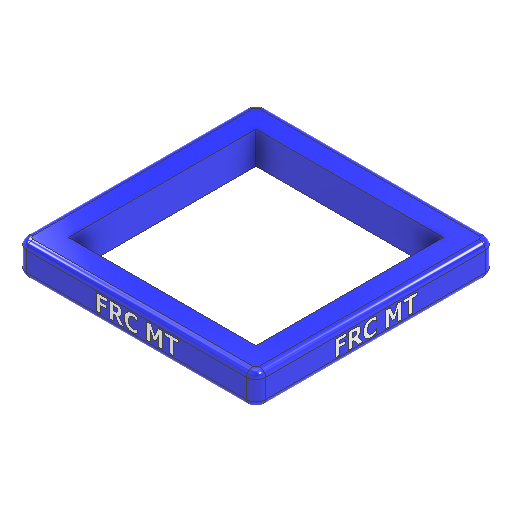
# Autodesk Inventor part: Bumper
Saved by Autodesk Inventor 2025.3 (Build 293356000, 356)
## iProperties
Created: 2026-05-15
Part Number: Bumper
Material: Genérico
Document SubType Name: Modeling
Designer: djair.oliveira
Density: 1 g/cm^3
Appearance: Padrão
Author: djair.oliveira
Autodesk Inventor part; units mm, degrees
ref_plane "YZ Plane" through (0, 0, 0) normal (1, 0, 0) x (0, 1, 0)
ref_plane "XZ Plane" through (0, 0, 0) normal (0, 1, 0) x (-1, 0, 0)
ref_plane "XY Plane" through (0, 0, 0) normal (0, 0, 1) x (1, 0, 0)
sketch "Esboço1" plane through (0, 0, 0) normal (0, 1, 0) x (-1, 0, 0)
  line L0 (-292.1, 292.1) -> (292.1, 292.1)
  line L1 (292.1, 292.1) -> (292.1, -292.1)
  line L2 (292.1, -292.1) -> (-292.1, -292.1)
  line L3 (-292.1, -292.1) -> (-292.1, 292.1)
  line L4 (-292.1, 292.1) -> (292.1, -292.1) construction
  line L5 (292.1, 292.1) -> (-292.1, -292.1) construction
  line L6 (-342.1, 372.1) -> (342.1, 372.1)
  line L7 (372.1, 342.1) -> (372.1, -342.1)
  line L8 (342.1, -372.1) -> (-342.1, -372.1)
  line L9 (-372.1, -342.1) -> (-372.1, 342.1)
  line L10 (-372.1, 372.1) -> (372.1, -372.1) construction
  line L11 (372.1, 372.1) -> (-372.1, -372.1) construction
  arc A0 (-372.1, -342.1) -> (-342.1, -372.1) centre (-342.1, -342.1) ccw
  arc A1 (-342.1, 372.1) -> (-372.1, 342.1) centre (-342.1, 342.1) ccw
  arc A2 (372.1, 342.1) -> (342.1, 372.1) centre (342.1, 342.1) ccw
  arc A3 (342.1, -372.1) -> (372.1, -342.1) centre (342.1, -342.1) ccw
  point P0 (0, 0)
  dimension "d0" = 584.2
  dimension "d1" = 584.2
  dimension "d2" = 80
  dimension "d3" = 30
  constraints: 24 end point, 9 point on line, 8 point on circle, 8 tangent, 4 centre point, 4 midpoint, 4 parallel, 3 equal radius, 2 horizontal, 2 perpendicular
  measures "d0" distance of L0.end L1.end
  measures "d1" distance of L1.end L2.end
  measures "d2" distance between parallel lines of L9 L3
  measures "d3" radius of A0
extrude "Extrusão1" add sketch "Esboço1" along normal blind 100
fillet "Arredondamento1" radius 20 16 edges at (363.3132, 100, -363.3132) (0, 100, -372.1) (-363.3132, 100, -363.3132) (-372.1, 100, 0) (-363.3132, 100, 363.3132) (0, 100, 372.1) (363.3132, 100, 363.3132) (372.1, 100, 0) (363.3132, 0, -363.3132) (0, 0, -372.1) (-363.3132, 0, -363.3132) (-372.1, 0, 0) (-363.3132, 0, 363.3132) (0, 0, 372.1) (363.3132, 0, 363.3132) (372.1, 0, 0)
sketch "Esboço2" plane through (372.1, 20, -342.1) normal (1, 0, 0) x (0, 0, -1)
  line L0 (-513.8978, 55) -> (-170.3022, 55) construction
  line L1 (-170.3022, 55) -> (-170.3022, 5) construction
  line L2 (-170.3022, 5) -> (-513.8978, 5) construction
  line L3 (-513.8978, 5) -> (-513.8978, 55) construction
  line L4 (30, 0) -> (30, 60) projected
  line L5 (-433.1859, 44.5057) -> (-454.1746, 44.5057)
  line L6 (-454.1746, 44.5057) -> (-454.1746, 35.0648)
  line L7 (-454.1746, 35.0648) -> (-434.8472, 35.0648)
  line L8 (-434.8472, 35.0648) -> (-434.8472, 25.5429)
  line L9 (-434.8472, 25.5429) -> (-454.1746, 25.5429)
  line L10 (-454.1746, 25.5429) -> (-454.1746, 4.0276)
  line L11 (-454.1746, 4.0276) -> (-466.6543, 4.0276)
  line L12 (-466.6543, 4.0276) -> (-466.6543, 54.0276)
  line L13 (-466.6543, 54.0276) -> (-433.1859, 54.0276)
  line L14 (-433.1859, 54.0276) -> (-433.1859, 44.5057)
  line L15 (-380.5117, 4.0276) -> (-395.7872, 4.0276)
  line L16 (-395.7872, 4.0276) -> (-409.6851, 22.3825)
  line L17 (-409.6851, 22.3825) -> (-414.2232, 22.3825)
  line L18 (-414.2232, 22.3825) -> (-414.2232, 4.0276)
  line L19 (-414.2232, 4.0276) -> (-426.7029, 4.0276)
  line L20 (-426.7029, 4.0276) -> (-426.7029, 54.0276)
  line L21 (-426.7029, 54.0276) -> (-406.6057, 54.0276)
  spline S0 degree 2 poles (-406.6057, 54.0276) (-402.4322, 54.0276) (-396.2734, 52.9741) (-393.6397, 51.3533) knots 0 0 0 1 2 2 2
  spline S1 degree 2 poles (-393.6397, 51.3533) (-390.9655, 49.6515) (-387.805, 44.3436) (-387.805, 40.2917) knots 0 0 0 1 2 2 2
  spline S2 degree 2 poles (-387.805, 40.2917) (-387.805, 34.5786) (-392.9914, 27.4068) (-397.3269, 25.2998) knots 0 0 0 1 2 2 2
  line L22 (-397.3269, 25.2998) -> (-380.5117, 4.0276)
  spline S3 degree 2 poles (-400.6899, 38.7115) (-400.6899, 40.6159) (-402.1486, 43.3306) (-403.8099, 44.06) knots 0 0 0 1 2 2 2
  spline S4 degree 2 poles (-403.8099, 44.06) (-404.9849, 44.5462) (-407.8617, 44.8298) (-410.0092, 44.8298) knots 0 0 0 1 2 2 2
  line L23 (-410.0092, 44.8298) -> (-414.2232, 44.8298)
  line L24 (-414.2232, 44.8298) -> (-414.2232, 31.3776)
  line L25 (-414.2232, 31.3776) -> (-410.617, 31.3776)
  spline S5 degree 2 poles (-410.617, 31.3776) (-408.0238, 31.3776) (-404.3366, 32.0259) (-403.0805, 33.0389) knots 0 0 0 1 2 2 2
  spline S6 degree 2 poles (-403.0805, 33.0389) (-401.865, 34.0113) (-400.6899, 36.6045) (-400.6899, 38.7115) knots 0 0 0 1 2 2 2
  spline S7 degree 2 poles (-355.228, 3.0551) (-366.4922, 3.0551) (-379.7013, 16.6694) (-379.7013, 28.987) knots 0 0 0 1 2 2 2
  spline S8 degree 2 poles (-379.7013, 28.987) (-379.7013, 40.859) (-366.4517, 55) (-355.1875, 55) knots 0 0 0 1 2 2 2
  spline S9 degree 2 poles (-355.1875, 55) (-352.2297, 55) (-347.4485, 54.3112) (-345.2604, 53.7439) knots 0 0 0 1 2 2 2
  spline S10 degree 2 poles (-345.2604, 53.7439) (-343.5587, 53.2172) (-339.5473, 51.4749) (-338.2912, 50.8266) knots 0 0 0 1 2 2 2
  line L26 (-338.2912, 50.8266) -> (-338.2912, 38.9141)
  line L27 (-338.2912, 38.9141) -> (-339.5473, 38.9141)
  spline S11 degree 2 poles (-339.5473, 38.9141) (-340.4793, 39.7245) (-343.2345, 41.9935) (-344.9768, 43.047) knots 0 0 0 1 2 2 2
  spline S12 degree 2 poles (-344.9768, 43.047) (-346.7191, 44.141) (-350.8925, 45.6402) (-353.2021, 45.6402) knots 0 0 0 1 2 2 2
  spline S13 degree 2 poles (-353.2021, 45.6402) (-355.9169, 45.6402) (-360.4144, 43.9384) (-362.4809, 41.7909) knots 0 0 0 1 2 2 2
  spline S14 degree 2 poles (-362.4809, 41.7909) (-364.3447, 39.8865) (-366.7353, 33.363) (-366.7353, 28.9465) knots 0 0 0 1 2 2 2
  spline S15 degree 2 poles (-366.7353, 28.9465) (-366.7353, 24.2869) (-364.2637, 17.9254) (-362.2378, 15.9806) knots 0 0 0 1 2 2 2
  spline S16 degree 2 poles (-362.2378, 15.9806) (-360.2929, 14.0762) (-355.5117, 12.4149) (-353.1211, 12.4149) knots 0 0 0 1 2 2 2
  spline S17 degree 2 poles (-353.1211, 12.4149) (-350.6494, 12.4149) (-346.1519, 14.0762) (-344.6122, 15.0891) knots 0 0 0 1 2 2 2
  spline S18 degree 2 poles (-344.6122, 15.0891) (-342.9104, 16.1021) (-340.3577, 18.2496) (-339.4258, 19.1005) knots 0 0 0 1 2 2 2
  line L28 (-339.4258, 19.1005) -> (-338.2912, 19.1005)
  line L29 (-338.2912, 19.1005) -> (-338.2912, 7.3501)
  spline S19 degree 2 poles (-338.2912, 7.3501) (-339.6689, 6.7018) (-343.275, 5.081) (-345.2199, 4.5138) knots 0 0 0 1 2 2 2
  spline S20 degree 2 poles (-345.2199, 4.5138) (-347.57, 3.7844) (-351.6624, 3.0551) (-355.228, 3.0551) knots 0 0 0 1 2 2 2
  line L30 (-259.6851, 4.0276) -> (-272.1648, 4.0276)
  line L31 (-272.1648, 4.0276) -> (-272.1648, 37.1718)
  line L32 (-272.1648, 37.1718) -> (-281.241, 15.778)
  line L33 (-281.241, 15.778) -> (-289.831, 15.778)
  line L34 (-289.831, 15.778) -> (-298.9071, 37.1718)
  line L35 (-298.9071, 37.1718) -> (-298.9071, 4.0276)
  line L36 (-298.9071, 4.0276) -> (-310.7386, 4.0276)
  line L37 (-310.7386, 4.0276) -> (-310.7386, 54.0276)
  line L38 (-310.7386, 54.0276) -> (-296.2734, 54.0276)
  line L39 (-296.2734, 54.0276) -> (-285.1713, 29.3517)
  line L40 (-285.1713, 29.3517) -> (-274.1502, 54.0276)
  line L41 (-274.1502, 54.0276) -> (-259.6851, 54.0276)
  line L42 (-259.6851, 54.0276) -> (-259.6851, 4.0276)
  line L43 (-239.7094, 4.0276) -> (-239.7094, 44.5057)
  line L44 (-239.7094, 44.5057) -> (-254.4987, 44.5057)
  line L45 (-254.4987, 44.5057) -> (-254.4987, 54.0276)
  line L46 (-254.4987, 54.0276) -> (-212.3593, 54.0276)
  line L47 (-212.3593, 54.0276) -> (-212.3593, 44.5057)
  line L48 (-212.3593, 44.5057) -> (-227.1486, 44.5057)
  line L49 (-227.1486, 44.5057) -> (-227.1486, 4.0276)
  line L50 (-227.1486, 4.0276) -> (-239.7094, 4.0276)
  point P0 (-342.1, -20)
  point P1 (-342.1, 55)
  point P2 (-170.3022, 30)
  point P3 (30, 30)
  dimension "d12" = 50
  constraints: 3 midpoint, 1 horizontal, 1 horizontal alignment, 1 vertical alignment, 2 other
  measures "d12" distance of L0.end L1.end
extrude "Extrusão2" cut sketch "Esboço2" against normal blind 0.1
sketch "Esboço3" plane through (342.1, 20, -372.1) normal (0, 0, -1) x (-1, 0, 0)
  line L0 (136.9103, 55) -> (547.2897, 55) construction
  line L1 (547.2897, 55) -> (547.2897, 5) construction
  line L2 (547.2897, 5) -> (136.9103, 5) construction
  line L3 (136.9103, 5) -> (136.9103, 55) construction
  line L4 (714.2, 0) -> (714.2, 60) projected
  line L5 (251.0141, 44.5057) -> (230.0254, 44.5057)
  line L6 (230.0254, 44.5057) -> (230.0254, 35.0648)
  line L7 (230.0254, 35.0648) -> (249.3528, 35.0648)
  line L8 (249.3528, 35.0648) -> (249.3528, 25.5429)
  line L9 (249.3528, 25.5429) -> (230.0254, 25.5429)
  line L10 (230.0254, 25.5429) -> (230.0254, 4.0276)
  line L11 (230.0254, 4.0276) -> (217.5457, 4.0276)
  line L12 (217.5457, 4.0276) -> (217.5457, 54.0276)
  line L13 (217.5457, 54.0276) -> (251.0141, 54.0276)
  line L14 (251.0141, 54.0276) -> (251.0141, 44.5057)
  line L15 (303.6883, 4.0276) -> (288.4128, 4.0276)
  line L16 (288.4128, 4.0276) -> (274.5149, 22.3825)
  line L17 (274.5149, 22.3825) -> (269.9768, 22.3825)
  line L18 (269.9768, 22.3825) -> (269.9768, 4.0276)
  line L19 (269.9768, 4.0276) -> (257.4971, 4.0276)
  line L20 (257.4971, 4.0276) -> (257.4971, 54.0276)
  line L21 (257.4971, 54.0276) -> (277.5943, 54.0276)
  spline S0 degree 2 poles (277.5943, 54.0276) (281.7678, 54.0276) (287.9266, 52.9741) (290.5603, 51.3533) knots 0 0 0 1 2 2 2
  spline S1 degree 2 poles (290.5603, 51.3533) (293.2345, 49.6515) (296.395, 44.3436) (296.395, 40.2917) knots 0 0 0 1 2 2 2
  spline S2 degree 2 poles (296.395, 40.2917) (296.395, 34.5786) (291.2086, 27.4068) (286.8731, 25.2998) knots 0 0 0 1 2 2 2
  line L22 (286.8731, 25.2998) -> (303.6883, 4.0276)
  spline S3 degree 2 poles (283.5101, 38.7115) (283.5101, 40.6159) (282.0514, 43.3306) (280.3901, 44.06) knots 0 0 0 1 2 2 2
  spline S4 degree 2 poles (280.3901, 44.06) (279.2151, 44.5462) (276.3383, 44.8298) (274.1908, 44.8298) knots 0 0 0 1 2 2 2
  line L23 (274.1908, 44.8298) -> (269.9768, 44.8298)
  line L24 (269.9768, 44.8298) -> (269.9768, 31.3776)
  line L25 (269.9768, 31.3776) -> (273.583, 31.3776)
  spline S5 degree 2 poles (273.583, 31.3776) (276.1762, 31.3776) (279.8634, 32.0259) (281.1195, 33.0389) knots 0 0 0 1 2 2 2
  spline S6 degree 2 poles (281.1195, 33.0389) (282.335, 34.0113) (283.5101, 36.6045) (283.5101, 38.7115) knots 0 0 0 1 2 2 2
  spline S7 degree 2 poles (328.972, 3.0551) (317.7078, 3.0551) (304.4987, 16.6694) (304.4987, 28.987) knots 0 0 0 1 2 2 2
  spline S8 degree 2 poles (304.4987, 28.987) (304.4987, 40.859) (317.7483, 55) (329.0125, 55) knots 0 0 0 1 2 2 2
  spline S9 degree 2 poles (329.0125, 55) (331.9703, 55) (336.7515, 54.3112) (338.9396, 53.7439) knots 0 0 0 1 2 2 2
  spline S10 degree 2 poles (338.9396, 53.7439) (340.6413, 53.2172) (344.6527, 51.4749) (345.9088, 50.8266) knots 0 0 0 1 2 2 2
  line L26 (345.9088, 50.8266) -> (345.9088, 38.9141)
  line L27 (345.9088, 38.9141) -> (344.6527, 38.9141)
  spline S11 degree 2 poles (344.6527, 38.9141) (343.7207, 39.7245) (340.9655, 41.9935) (339.2232, 43.047) knots 0 0 0 1 2 2 2
  spline S12 degree 2 poles (339.2232, 43.047) (337.4809, 44.141) (333.3075, 45.6402) (330.9979, 45.6402) knots 0 0 0 1 2 2 2
  spline S13 degree 2 poles (330.9979, 45.6402) (328.2831, 45.6402) (323.7856, 43.9384) (321.7191, 41.7909) knots 0 0 0 1 2 2 2
  spline S14 degree 2 poles (321.7191, 41.7909) (319.8553, 39.8865) (317.4647, 33.363) (317.4647, 28.9465) knots 0 0 0 1 2 2 2
  spline S15 degree 2 poles (317.4647, 28.9465) (317.4647, 24.2869) (319.9363, 17.9254) (321.9622, 15.9806) knots 0 0 0 1 2 2 2
  spline S16 degree 2 poles (321.9622, 15.9806) (323.9071, 14.0762) (328.6883, 12.4149) (331.0789, 12.4149) knots 0 0 0 1 2 2 2
  spline S17 degree 2 poles (331.0789, 12.4149) (333.5506, 12.4149) (338.0481, 14.0762) (339.5878, 15.0891) knots 0 0 0 1 2 2 2
  spline S18 degree 2 poles (339.5878, 15.0891) (341.2896, 16.1021) (343.8423, 18.2496) (344.7742, 19.1005) knots 0 0 0 1 2 2 2
  line L28 (344.7742, 19.1005) -> (345.9088, 19.1005)
  line L29 (345.9088, 19.1005) -> (345.9088, 7.3501)
  spline S19 degree 2 poles (345.9088, 7.3501) (344.5311, 6.7018) (340.925, 5.081) (338.9801, 4.5138) knots 0 0 0 1 2 2 2
  spline S20 degree 2 poles (338.9801, 4.5138) (336.63, 3.7844) (332.5376, 3.0551) (328.972, 3.0551) knots 0 0 0 1 2 2 2
  line L30 (424.5149, 4.0276) -> (412.0352, 4.0276)
  line L31 (412.0352, 4.0276) -> (412.0352, 37.1718)
  line L32 (412.0352, 37.1718) -> (402.959, 15.778)
  line L33 (402.959, 15.778) -> (394.369, 15.778)
  line L34 (394.369, 15.778) -> (385.2929, 37.1718)
  line L35 (385.2929, 37.1718) -> (385.2929, 4.0276)
  line L36 (385.2929, 4.0276) -> (373.4614, 4.0276)
  line L37 (373.4614, 4.0276) -> (373.4614, 54.0276)
  line L38 (373.4614, 54.0276) -> (387.9266, 54.0276)
  line L39 (387.9266, 54.0276) -> (399.0287, 29.3517)
  line L40 (399.0287, 29.3517) -> (410.0498, 54.0276)
  line L41 (410.0498, 54.0276) -> (424.5149, 54.0276)
  line L42 (424.5149, 54.0276) -> (424.5149, 4.0276)
  line L43 (444.4906, 4.0276) -> (444.4906, 44.5057)
  line L44 (444.4906, 44.5057) -> (429.7013, 44.5057)
  line L45 (429.7013, 44.5057) -> (429.7013, 54.0276)
  line L46 (429.7013, 54.0276) -> (471.8407, 54.0276)
  line L47 (471.8407, 54.0276) -> (471.8407, 44.5057)
  line L48 (471.8407, 44.5057) -> (457.0514, 44.5057)
  line L49 (457.0514, 44.5057) -> (457.0514, 4.0276)
  line L50 (457.0514, 4.0276) -> (444.4906, 4.0276)
  point P0 (342.1, -20)
  point P1 (342.1, 55)
  point P2 (547.2897, 30)
  point P3 (714.2, 30)
  dimension "d9" = 50
  constraints: 3 midpoint, 1 horizontal alignment, 1 vertical alignment, 2 other
  measures "d9" distance of L0.end L1.end
extrude "Extrusão3" cut sketch "Esboço3" against normal blind 0.1
sketch "Esboço4" plane through (-342.1, 20, 372.1) normal (0, 0, 1) x (1, 0, 0)
  line L0 (96.734, 55.9724) -> (587.466, 55.9724) construction
  line L1 (587.466, 55.9724) -> (587.466, 4.0276) construction
  line L2 (587.466, 4.0276) -> (96.734, 4.0276) construction
  line L3 (96.734, 4.0276) -> (96.734, 55.9724) construction
  line L4 (714.2, 0) -> (714.2, 60) projected
  line L5 (251.0141, 45.4781) -> (230.0254, 45.4781)
  line L6 (230.0254, 45.4781) -> (230.0254, 36.0373)
  line L7 (230.0254, 36.0373) -> (249.3528, 36.0373)
  line L8 (249.3528, 36.0373) -> (249.3528, 26.5154)
  line L9 (249.3528, 26.5154) -> (230.0254, 26.5154)
  line L10 (230.0254, 26.5154) -> (230.0254, 5)
  line L11 (230.0254, 5) -> (217.5457, 5)
  line L12 (217.5457, 5) -> (217.5457, 55)
  line L13 (217.5457, 55) -> (251.0141, 55)
  line L14 (251.0141, 55) -> (251.0141, 45.4781)
  line L15 (303.6883, 5) -> (288.4128, 5)
  line L16 (288.4128, 5) -> (274.5149, 23.3549)
  line L17 (274.5149, 23.3549) -> (269.9768, 23.3549)
  line L18 (269.9768, 23.3549) -> (269.9768, 5)
  line L19 (269.9768, 5) -> (257.4971, 5)
  line L20 (257.4971, 5) -> (257.4971, 55)
  line L21 (257.4971, 55) -> (277.5943, 55)
  spline S0 degree 2 poles (277.5943, 55) (281.7678, 55) (287.9266, 53.9465) (290.5603, 52.3258) knots 0 0 0 1 2 2 2
  spline S1 degree 2 poles (290.5603, 52.3258) (293.2345, 50.624) (296.395, 45.316) (296.395, 41.2642) knots 0 0 0 1 2 2 2
  spline S2 degree 2 poles (296.395, 41.2642) (296.395, 35.5511) (291.2086, 28.3793) (286.8731, 26.2723) knots 0 0 0 1 2 2 2
  line L22 (286.8731, 26.2723) -> (303.6883, 5)
  spline S3 degree 2 poles (283.5101, 39.684) (283.5101, 41.5883) (282.0514, 44.3031) (280.3901, 45.0324) knots 0 0 0 1 2 2 2
  spline S4 degree 2 poles (280.3901, 45.0324) (279.2151, 45.5186) (276.3383, 45.8023) (274.1908, 45.8023) knots 0 0 0 1 2 2 2
  line L23 (274.1908, 45.8023) -> (269.9768, 45.8023)
  line L24 (269.9768, 45.8023) -> (269.9768, 32.3501)
  line L25 (269.9768, 32.3501) -> (273.583, 32.3501)
  spline S5 degree 2 poles (273.583, 32.3501) (276.1762, 32.3501) (279.8634, 32.9984) (281.1195, 34.0113) knots 0 0 0 1 2 2 2
  spline S6 degree 2 poles (281.1195, 34.0113) (282.335, 34.9838) (283.5101, 37.577) (283.5101, 39.684) knots 0 0 0 1 2 2 2
  spline S7 degree 2 poles (328.972, 4.0276) (317.7078, 4.0276) (304.4987, 17.6418) (304.4987, 29.9595) knots 0 0 0 1 2 2 2
  spline S8 degree 2 poles (304.4987, 29.9595) (304.4987, 41.8314) (317.7483, 55.9724) (329.0125, 55.9724) knots 0 0 0 1 2 2 2
  spline S9 degree 2 poles (329.0125, 55.9724) (331.9703, 55.9724) (336.7515, 55.2836) (338.9396, 54.7164) knots 0 0 0 1 2 2 2
  spline S10 degree 2 poles (338.9396, 54.7164) (340.6413, 54.1896) (344.6527, 52.4473) (345.9088, 51.799) knots 0 0 0 1 2 2 2
  line L26 (345.9088, 51.799) -> (345.9088, 39.8865)
  line L27 (345.9088, 39.8865) -> (344.6527, 39.8865)
  spline S11 degree 2 poles (344.6527, 39.8865) (343.7207, 40.6969) (340.9655, 42.966) (339.2232, 44.0194) knots 0 0 0 1 2 2 2
  spline S12 degree 2 poles (339.2232, 44.0194) (337.4809, 45.1135) (333.3075, 46.6126) (330.9979, 46.6126) knots 0 0 0 1 2 2 2
  spline S13 degree 2 poles (330.9979, 46.6126) (328.2831, 46.6126) (323.7856, 44.9109) (321.7191, 42.7634) knots 0 0 0 1 2 2 2
  spline S14 degree 2 poles (321.7191, 42.7634) (319.8553, 40.859) (317.4647, 34.3355) (317.4647, 29.919) knots 0 0 0 1 2 2 2
  spline S15 degree 2 poles (317.4647, 29.919) (317.4647, 25.2593) (319.9363, 18.8979) (321.9622, 16.953) knots 0 0 0 1 2 2 2
  spline S16 degree 2 poles (321.9622, 16.953) (323.9071, 15.0486) (328.6883, 13.3874) (331.0789, 13.3874) knots 0 0 0 1 2 2 2
  spline S17 degree 2 poles (331.0789, 13.3874) (333.5506, 13.3874) (338.0481, 15.0486) (339.5878, 16.0616) knots 0 0 0 1 2 2 2
  spline S18 degree 2 poles (339.5878, 16.0616) (341.2896, 17.0746) (343.8423, 19.222) (344.7742, 20.0729) knots 0 0 0 1 2 2 2
  line L28 (344.7742, 20.0729) -> (345.9088, 20.0729)
  line L29 (345.9088, 20.0729) -> (345.9088, 8.3225)
  spline S19 degree 2 poles (345.9088, 8.3225) (344.5311, 7.6742) (340.925, 6.0535) (338.9801, 5.4862) knots 0 0 0 1 2 2 2
  spline S20 degree 2 poles (338.9801, 5.4862) (336.63, 4.7569) (332.5376, 4.0276) (328.972, 4.0276) knots 0 0 0 1 2 2 2
  line L30 (424.5149, 5) -> (412.0352, 5)
  line L31 (412.0352, 5) -> (412.0352, 38.1442)
  line L32 (412.0352, 38.1442) -> (402.959, 16.7504)
  line L33 (402.959, 16.7504) -> (394.369, 16.7504)
  line L34 (394.369, 16.7504) -> (385.2929, 38.1442)
  line L35 (385.2929, 38.1442) -> (385.2929, 5)
  line L36 (385.2929, 5) -> (373.4614, 5)
  line L37 (373.4614, 5) -> (373.4614, 55)
  line L38 (373.4614, 55) -> (387.9266, 55)
  line L39 (387.9266, 55) -> (399.0287, 30.3241)
  line L40 (399.0287, 30.3241) -> (410.0498, 55)
  line L41 (410.0498, 55) -> (424.5149, 55)
  line L42 (424.5149, 55) -> (424.5149, 5)
  line L43 (444.4906, 5) -> (444.4906, 45.4781)
  line L44 (444.4906, 45.4781) -> (429.7013, 45.4781)
  line L45 (429.7013, 45.4781) -> (429.7013, 55)
  line L46 (429.7013, 55) -> (471.8407, 55)
  line L47 (471.8407, 55) -> (471.8407, 45.4781)
  line L48 (471.8407, 45.4781) -> (457.0514, 45.4781)
  line L49 (457.0514, 45.4781) -> (457.0514, 5)
  line L50 (457.0514, 5) -> (444.4906, 5)
  point P0 (342.1, -20)
  point P1 (587.466, 30)
  point P2 (714.2, 30)
  point P3 (342.1, 55.9724)
  constraints: 3 midpoint, 1 horizontal, 1 horizontal alignment, 1 vertical alignment, 2 other
extrude "Extrusão4" cut sketch "Esboço4" against normal blind 0.1
sketch "Esboço5" plane through (-372.1, 20, 342.1) normal (-1, 0, 0) x (0, 0, 1)
  line L0 (-621.9565, 55.9724) -> (-62.2435, 55.9724) construction
  line L1 (-62.2435, 55.9724) -> (-62.2435, 4.0276) construction
  line L2 (-62.2435, 4.0276) -> (-621.9565, 4.0276) construction
  line L3 (-621.9565, 4.0276) -> (-621.9565, 55.9724) construction
  line L4 (30, 0) -> (30, 60) projected
  line L5 (-433.1859, 45.4781) -> (-454.1746, 45.4781)
  line L6 (-454.1746, 45.4781) -> (-454.1746, 36.0373)
  line L7 (-454.1746, 36.0373) -> (-434.8472, 36.0373)
  line L8 (-434.8472, 36.0373) -> (-434.8472, 26.5154)
  line L9 (-434.8472, 26.5154) -> (-454.1746, 26.5154)
  line L10 (-454.1746, 26.5154) -> (-454.1746, 5)
  line L11 (-454.1746, 5) -> (-466.6543, 5)
  line L12 (-466.6543, 5) -> (-466.6543, 55)
  line L13 (-466.6543, 55) -> (-433.1859, 55)
  line L14 (-433.1859, 55) -> (-433.1859, 45.4781)
  line L15 (-380.5117, 5) -> (-395.7872, 5)
  line L16 (-395.7872, 5) -> (-409.6851, 23.3549)
  line L17 (-409.6851, 23.3549) -> (-414.2232, 23.3549)
  line L18 (-414.2232, 23.3549) -> (-414.2232, 5)
  line L19 (-414.2232, 5) -> (-426.7029, 5)
  line L20 (-426.7029, 5) -> (-426.7029, 55)
  line L21 (-426.7029, 55) -> (-406.6057, 55)
  spline S0 degree 2 poles (-406.6057, 55) (-402.4322, 55) (-396.2734, 53.9465) (-393.6397, 52.3258) knots 0 0 0 1 2 2 2
  spline S1 degree 2 poles (-393.6397, 52.3258) (-390.9655, 50.624) (-387.805, 45.316) (-387.805, 41.2642) knots 0 0 0 1 2 2 2
  spline S2 degree 2 poles (-387.805, 41.2642) (-387.805, 35.5511) (-392.9914, 28.3793) (-397.3269, 26.2723) knots 0 0 0 1 2 2 2
  line L22 (-397.3269, 26.2723) -> (-380.5117, 5)
  spline S3 degree 2 poles (-400.6899, 39.684) (-400.6899, 41.5883) (-402.1486, 44.3031) (-403.8099, 45.0324) knots 0 0 0 1 2 2 2
  spline S4 degree 2 poles (-403.8099, 45.0324) (-404.9849, 45.5186) (-407.8617, 45.8023) (-410.0092, 45.8023) knots 0 0 0 1 2 2 2
  line L23 (-410.0092, 45.8023) -> (-414.2232, 45.8023)
  line L24 (-414.2232, 45.8023) -> (-414.2232, 32.3501)
  line L25 (-414.2232, 32.3501) -> (-410.617, 32.3501)
  spline S5 degree 2 poles (-410.617, 32.3501) (-408.0238, 32.3501) (-404.3366, 32.9984) (-403.0805, 34.0113) knots 0 0 0 1 2 2 2
  spline S6 degree 2 poles (-403.0805, 34.0113) (-401.865, 34.9838) (-400.6899, 37.577) (-400.6899, 39.684) knots 0 0 0 1 2 2 2
  spline S7 degree 2 poles (-355.228, 4.0276) (-366.4922, 4.0276) (-379.7013, 17.6418) (-379.7013, 29.9595) knots 0 0 0 1 2 2 2
  spline S8 degree 2 poles (-379.7013, 29.9595) (-379.7013, 41.8314) (-366.4517, 55.9724) (-355.1875, 55.9724) knots 0 0 0 1 2 2 2
  spline S9 degree 2 poles (-355.1875, 55.9724) (-352.2297, 55.9724) (-347.4485, 55.2836) (-345.2604, 54.7164) knots 0 0 0 1 2 2 2
  spline S10 degree 2 poles (-345.2604, 54.7164) (-343.5587, 54.1896) (-339.5473, 52.4473) (-338.2912, 51.799) knots 0 0 0 1 2 2 2
  line L26 (-338.2912, 51.799) -> (-338.2912, 39.8865)
  line L27 (-338.2912, 39.8865) -> (-339.5473, 39.8865)
  spline S11 degree 2 poles (-339.5473, 39.8865) (-340.4793, 40.6969) (-343.2345, 42.966) (-344.9768, 44.0194) knots 0 0 0 1 2 2 2
  spline S12 degree 2 poles (-344.9768, 44.0194) (-346.7191, 45.1135) (-350.8925, 46.6126) (-353.2021, 46.6126) knots 0 0 0 1 2 2 2
  spline S13 degree 2 poles (-353.2021, 46.6126) (-355.9169, 46.6126) (-360.4144, 44.9109) (-362.4809, 42.7634) knots 0 0 0 1 2 2 2
  spline S14 degree 2 poles (-362.4809, 42.7634) (-364.3447, 40.859) (-366.7353, 34.3355) (-366.7353, 29.919) knots 0 0 0 1 2 2 2
  spline S15 degree 2 poles (-366.7353, 29.919) (-366.7353, 25.2593) (-364.2637, 18.8979) (-362.2378, 16.953) knots 0 0 0 1 2 2 2
  spline S16 degree 2 poles (-362.2378, 16.953) (-360.2929, 15.0486) (-355.5117, 13.3874) (-353.1211, 13.3874) knots 0 0 0 1 2 2 2
  spline S17 degree 2 poles (-353.1211, 13.3874) (-350.6494, 13.3874) (-346.1519, 15.0486) (-344.6122, 16.0616) knots 0 0 0 1 2 2 2
  spline S18 degree 2 poles (-344.6122, 16.0616) (-342.9104, 17.0746) (-340.3577, 19.222) (-339.4258, 20.0729) knots 0 0 0 1 2 2 2
  line L28 (-339.4258, 20.0729) -> (-338.2912, 20.0729)
  line L29 (-338.2912, 20.0729) -> (-338.2912, 8.3225)
  spline S19 degree 2 poles (-338.2912, 8.3225) (-339.6689, 7.6742) (-343.275, 6.0535) (-345.2199, 5.4862) knots 0 0 0 1 2 2 2
  spline S20 degree 2 poles (-345.2199, 5.4862) (-347.57, 4.7569) (-351.6624, 4.0276) (-355.228, 4.0276) knots 0 0 0 1 2 2 2
  line L30 (-259.6851, 5) -> (-272.1648, 5)
  line L31 (-272.1648, 5) -> (-272.1648, 38.1442)
  line L32 (-272.1648, 38.1442) -> (-281.241, 16.7504)
  line L33 (-281.241, 16.7504) -> (-289.831, 16.7504)
  line L34 (-289.831, 16.7504) -> (-298.9071, 38.1442)
  line L35 (-298.9071, 38.1442) -> (-298.9071, 5)
  line L36 (-298.9071, 5) -> (-310.7386, 5)
  line L37 (-310.7386, 5) -> (-310.7386, 55)
  line L38 (-310.7386, 55) -> (-296.2734, 55)
  line L39 (-296.2734, 55) -> (-285.1713, 30.3241)
  line L40 (-285.1713, 30.3241) -> (-274.1502, 55)
  line L41 (-274.1502, 55) -> (-259.6851, 55)
  line L42 (-259.6851, 55) -> (-259.6851, 5)
  line L43 (-239.7094, 5) -> (-239.7094, 45.4781)
  line L44 (-239.7094, 45.4781) -> (-254.4987, 45.4781)
  line L45 (-254.4987, 45.4781) -> (-254.4987, 55)
  line L46 (-254.4987, 55) -> (-212.3593, 55)
  line L47 (-212.3593, 55) -> (-212.3593, 45.4781)
  line L48 (-212.3593, 45.4781) -> (-227.1486, 45.4781)
  line L49 (-227.1486, 45.4781) -> (-227.1486, 5)
  line L50 (-227.1486, 5) -> (-239.7094, 5)
  point P0 (-342.1, -20)
  point P1 (-62.2435, 30)
  point P2 (30, 30)
  point P3 (-342.1, 55.9724)
  constraints: 3 midpoint, 1 horizontal, 1 horizontal alignment, 1 vertical alignment, 2 other
extrude "Extrusão5" cut sketch "Esboço5" against normal blind 0.1
equation "\"d1\" = d0"
